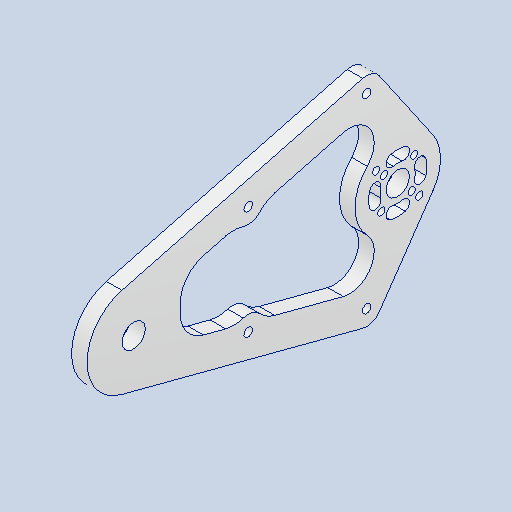
# Autodesk Inventor part: Frame (Motor Side)
Saved by Autodesk Inventor 2022.3 (Build 263350000, 350)
## iProperties
Created: 2022-05-22
Part Number: Frame (Motor Side)
Material: Aluminum 6061
Document SubType Name: Modeling
Designer: Nathan Cai
Density: 2.7 g/cm^3
Appearance: Aluminum - Flat
Mass: 82.1792 g
Surface Area: 150.773 cm^2
Volume: 30.4368 cm^3
Author: Nathan Cai
Autodesk Inventor part; units mm, degrees
ref_plane "YZ Plane" through (0, 0, 0) normal (1, 0, 0) x (0, 1, 0)
ref_plane "XZ Plane" through (0, 0, 0) normal (0, 1, 0) x (-1, 0, 0)
ref_plane "XY Plane" through (0, 0, 0) normal (0, 0, 1) x (1, 0, 0)
sketch "Sketch1" plane through (0, 0, 0) normal (1, 0, 0) x (0, 1, 0)
  circle A0 centre (0, 0) radius 4.7625
  circle A1 centre (0, 0) radius 17.4625
  line L0 (0, 0) -> (0, 107.95) construction
  circle A2 centre (0, 107.95) radius 4.7625
  circle A3 centre (0, 107.95) radius 76.2 construction
  circle A4 centre (0, 107.95) radius 19.05
  line L1 (0, 12.7) -> (38.1, 12.7) construction
  circle A5 centre (38.1, 12.7) radius 1.7526
  arc A6 (31.9576, 11.0897) -> (34.5035, 17.9333) centre (38.1, 12.7) ccw
  line L2 (41.6965, 7.4667) -> (9.8904, -14.3916)
  line L3 (18.4273, 112.7809) -> (44.2424, 14.3103)
  line L4 (10.6971, 92.1869) -> (31.9576, 11.0897)
  line L5 (34.5035, 17.9333) -> (16.5434, 5.5905) construction
  circle A7 centre (-38.1, 12.7) radius 1.7526
  arc A8 (-34.5035, 17.9333) -> (-31.9576, 11.0897) centre (-38.1, 12.7) ccw
  line L6 (-41.6965, 7.4667) -> (-9.8904, -14.3916)
  line L7 (-18.4273, 112.7809) -> (-44.2424, 14.3103)
  line L8 (-10.6971, 92.1869) -> (-31.9576, 11.0897)
  line L9 (-34.5035, 17.9333) -> (-16.5434, 5.5905)
  line L10 (0, 0) -> (9.5, 0) construction
  line L11 (0, 0) -> (12.7, 0) construction
  line L12 (38.1, 12.7) -> (15.8856, 97.4357) construction
  circle A9 centre (25.4, 61.1435) radius 1.7526
  circle A10 centre (-25.4, 61.1435) radius 1.7526
  arc A11 (12.2057, 12.4884) -> (29.027, 22.2681) centre (19.2619, 19.708) ccw
  arc A12 (-29.027, 22.2681) -> (-12.2057, 12.4884) centre (-19.2619, 19.708) ccw
  line L13 (0, 0) -> (6.7175, -6.7175) construction
  line L14 (0, 0) -> (9.5, 0) construction
  line L15 (0, 0) -> (5.6569, 5.6569) construction
  circle A13 centre (6.7175, -6.7175) radius 1.5
  circle A14 centre (5.6569, 5.6569) radius 1.5
  arc A15 (9.2004, -2.4653) -> (9.2004, 2.4653) centre (0, 0) ccw construction
  arc A16 (11.5006, -3.0816) -> (11.5006, 3.0816) centre (0, 0) ccw
  arc A17 (6.9003, -1.8489) -> (6.9003, 1.8489) centre (0, 0) ccw
  arc A18 (6.9003, -1.8489) -> (11.5006, -3.0816) centre (9.2004, -2.4653) ccw
  arc A19 (11.5006, 3.0816) -> (6.9003, 1.8489) centre (9.2004, 2.4653) ccw
  line L16 (0, 0) -> (9.2004, -2.4653) construction
  line L17 (0, 0) -> (9.525, 0) construction
  line L18 (0, 0) -> (9.2004, 2.4653) construction
  arc A20 (3.0816, 11.5006) -> (-3.0816, 11.5006) centre (0, 0) ccw
  arc A21 (2.4653, 9.2004) -> (-2.4653, 9.2004) centre (0, 0) ccw construction
  arc A22 (1.8489, 6.9003) -> (-1.8489, 6.9003) centre (0, 0) ccw
  arc A23 (-3.0816, 11.5006) -> (-1.8489, 6.9003) centre (-2.4653, 9.2004) ccw
  arc A24 (1.8489, 6.9003) -> (3.0816, 11.5006) centre (2.4653, 9.2004) ccw
  arc A25 (-11.5006, 3.0816) -> (-11.5006, -3.0816) centre (0, 0) ccw
  arc A26 (-9.2004, 2.4653) -> (-9.2004, -2.4653) centre (0, 0) ccw construction
  arc A27 (-6.9003, 1.8489) -> (-6.9003, -1.8489) centre (0, 0) ccw
  arc A28 (-11.5006, -3.0816) -> (-6.9003, -1.8489) centre (-9.2004, -2.4653) ccw
  arc A29 (-6.9003, 1.8489) -> (-11.5006, 3.0816) centre (-9.2004, 2.4653) ccw
  arc A30 (-3.0816, -11.5006) -> (3.0816, -11.5006) centre (0, 0) ccw
  arc A31 (-2.4653, -9.2004) -> (2.4653, -9.2004) centre (0, 0) ccw construction
  arc A32 (-1.8489, -6.9003) -> (1.8489, -6.9003) centre (0, 0) ccw
  arc A33 (3.0816, -11.5006) -> (1.8489, -6.9003) centre (2.4653, -9.2004) ccw
  arc A34 (-1.8489, -6.9003) -> (-3.0816, -11.5006) centre (-2.4653, -9.2004) ccw
  line L19 (0, 0) -> (8.8388, 8.8388) construction
  circle A35 centre (8.8388, 8.8388) radius 1.5
  circle A36 centre (-5.6569, -5.6569) radius 1.5
  circle A37 centre (-6.7175, 6.7175) radius 1.5
  circle A38 centre (-8.8388, -8.8388) radius 1.5
  line L20 (25.4, 61.1435) -> (-25.4, 61.1435) construction
  circle A39 centre (22.225, 61.1435) radius 6.35
  circle A40 centre (22.225, 61.1435) radius 1.7526
  circle A41 centre (-22.225, 61.1435) radius 6.35
  circle A42 centre (-22.225, 61.1435) radius 1.7526
  point P0 (-18.4273, 112.7809)
  point P1 (-9.8904, -14.3916)
  point P2 (30.826, 15.406)
  point P3 (-16.5434, 5.5905)
  point P4 (-30.826, 15.406)
  point P5 (-29.027, 22.2681)
  point P6 (0, 9.525)
  point P7 (0, 9.5)
  point P8 (0, 12.7)
  point P9 (0, 9.5)
  point P10 (-9.525, 0)
  point P11 (-9.5, 0)
  point P12 (-12.7, 0)
  point P13 (-9.5, 0)
  point P14 (0, -9.525)
  point P15 (0, -9.5)
  point P16 (0, -12.7)
  point P17 (0, -9.5)
  point P18 (17.6744, 65.5723)
  point P19 (20.4324, 55.0518)
  point P20 (-20.4324, 55.0518)
  point P21 (-17.6744, 65.5723)
  dimension "d0" = 9.525
  dimension "d1" = 34.925
  dimension "d2" = 107.95
  dimension "d3" = 9.525
  dimension "d4" = 152.4
  dimension "d5" = 38.1
  dimension "d6" = 38.1
  dimension "d7" = 3.5052
  dimension "d8" = 12.7
  dimension "d9" = 12.7
  dimension "d10" = 12.7
  dimension "d11" = 12.7
  dimension "d36" = 3.5052
  dimension "d37" = 25.4
  dimension "d54" = 9.5
  dimension "d55" = 45
  dimension "d56" = 8
  dimension "d57" = 3
  dimension "d58" = 3
  dimension "d59" = 9.525
  dimension "d60" = 15
  dimension "d61" = 30
  dimension "d62" = 4.7625
  dimension "d65" = 360
  dimension "d67" = 12.5
  dimension "d68" = 3
  dimension "d71" = 360
  dimension "d73" = 12.7
  dimension "d74" = 3.5052
  dimension "d75" = 22.225
  constraints: 58 point on circle, 43 centre point, 42 end point, 17 symmetric about line, 16 coincident, 11 tangent, 6 horizontal, 4 point on line, 3 parallel, 2 equal length, 1 collinear, 1 perpendicular, 1 vertical, 84 other
  measures "d0" diameter of A0
  measures "d1" diameter of A1
  measures "d2" distance of L0.start L0.end
  measures "d3" diameter of A2
  measures "d4" diameter of A3
  measures "d5" diameter of A4
  measures "d6" distance of L1.start L1.end
  measures "d7" diameter of A5
  measures "d8" diameter of A6
  measures "d9" distance from line of A0.centre L1
  measures "d10" distance between parallel lines of L3 L4
  measures "d11" distance between parallel lines of L2 L5
  measures "d36" diameter of A9
  measures "d37" distance from line of L0 L20.start
  measures "d54" distance of L11.start L13.end
  measures "d55" angle of L13 L14
  measures "d56" distance of L11.start L15.end
  measures "d57" diameter of A13
  measures "d58" diameter of A14
  measures "d59" radius of A15
  measures "d60" angle of L16 L17
  measures "d61" angle of L16 L18
  measures "d62" diameter of A19
  measures "d67" distance of L19.start L19.end
  measures "d68" diameter of A35
  measures "d73" diameter of A39
  measures "d74" diameter of A40
  measures "d75" distance from line of L0 A40.centre
extrude "Extrusion1" add sketch "Sketch1" along normal blind 6.35 contours A1 | A1 A11 L4 A6 L2 | A1 L9 A12 | L4 A39 A4 L3 A6 | L6 A8 L8 L9 A1 | L9 L8 A12 | A39 L4 | L4 A39 | A8 L9 L8 | L9 A8 L7 A4 L8 A41 | A4 | A41 L8 | L8 A41 | A9 A40 | A42 A10 picked at (26.0767, 61.2857) picked at (-26.0767, 61.2857)
fillet "Fillet1" radius 12.7 6 edges at (3.175, 10.6971, 92.1869) (3.175, -10.6971, 92.1869) (3.175, 17.6744, 65.5723) (3.175, 20.4324, 55.0518) (3.175, -20.4324, 55.0518) (3.175, -17.6744, 65.5723)
equation "\"d10\" = d8"
equation "\"d11\" = d10"
body "Solid1"
